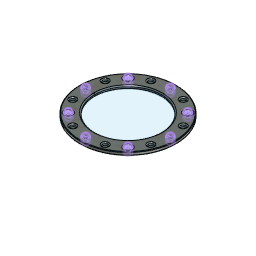
80mm-Gasket (Autodesk Fusion 360 design; units mm, degrees)
Autodesk Fusion 360 part; units mm, degrees
note: some values were not read from the file. Set by a fixed rule: which sketch regions a step uses.
sketch "Sketch1" plane through (0, 0, -3) normal (0, 0, -1) x (1, 0, 0)
  circle A0 centre (0, 0) radius 57.9733
  arc A1 (-37.591, -37.591) -> (-34.409, -34.409) centre (-36, -36) ccw
  arc A2 (-37.591, 37.591) -> (-34.409, 34.409) centre (-36, 36) ccw
  arc A3 (37.591, 37.591) -> (34.409, 34.409) centre (36, 36) ccw
  arc A4 (37.591, -37.591) -> (34.409, -34.409) centre (36, -36) ccw
  spline S0 degree 3 poles (-40, 0) (-40, -6.463) (-38.4036, -12.9202) (-32.3924, -24.3347) (-27.9941, -29.2878) (-18.5638, -35.7844) (-13.8953, -37.8426) (-2.3688, -40.5075) (4.666, -40.3075) (14.8449, -37.3359) (18.3282, -35.755) (26.9944, -30.2237) (31.596, -25.3745) (37.2725, -15.3601) (38.9152, -10.5255) (40.5307, 0.9912) (39.7923, 7.7648) (35.8254, 18.4158) (33.3642, 22.5705) (26.205, 30.8483) (21.0525, 34.5704) (10.4898, 38.9549) (5.2459, 40) (-6.442, 40) (-12.8781, 38.4142) (-23.2056, 32.9962) (-27.346, 29.6555) (-34.0803, 21.597) (-36.6527, 16.8665) (-39.3955, 7.9995) (-40, 4) (-40, 0) knots -1 -1 -1 -1 -0.922853 -0.922853 -0.84601 -0.84601 -0.786161 -0.786161 -0.704794 -0.704794 -0.659587 -0.659587 -0.582074 -0.582074 -0.522181 -0.522181 -0.443257 -0.443257 -0.386513 -0.386513 -0.312619 -0.312619 -0.25 -0.25 -0.173105 -0.173105 -0.11079 -0.11079 -0.047746 -0.047746 0 0 0 0
  circle A5 centre (0, 0) radius 57.9733
  spline S1 degree 3 poles (-40, 0) (-40, -6.463) (-38.4036, -12.9202) (-32.3924, -24.3347) (-27.9941, -29.2878) (-18.5638, -35.7844) (-13.8953, -37.8426) (-2.3688, -40.5075) (4.666, -40.3075) (14.8449, -37.3359) (18.3282, -35.755) (26.9944, -30.2237) (31.596, -25.3745) (37.2725, -15.3601) (38.9152, -10.5255) (40.5307, 0.9912) (39.7923, 7.7648) (35.8254, 18.4158) (33.3642, 22.5705) (26.205, 30.8483) (21.0525, 34.5704) (10.4898, 38.9549) (5.2459, 40) (-6.442, 40) (-12.8781, 38.4142) (-23.2056, 32.9962) (-27.346, 29.6555) (-34.0803, 21.597) (-36.6527, 16.8665) (-39.3955, 7.9995) (-40, 4) (-40, 0) knots -1 -1 -1 -1 -0.922853 -0.922853 -0.84601 -0.84601 -0.786161 -0.786161 -0.704794 -0.704794 -0.659587 -0.659587 -0.582074 -0.582074 -0.522181 -0.522181 -0.443257 -0.443257 -0.386513 -0.386513 -0.312619 -0.312619 -0.25 -0.25 -0.173105 -0.173105 -0.11079 -0.11079 -0.047746 -0.047746 0 0 0 0
  arc A6 (-37.591, 37.591) -> (-34.409, 34.409) centre (-36, 36) ccw construction
  arc A7 (37.591, 37.591) -> (34.409, 34.409) centre (36, 36) ccw construction
  circle A8 centre (36, -36) radius 2.1 construction
  arc A9 (-37.591, -37.591) -> (-34.409, -34.409) centre (-36, -36) ccw construction
  circle A10 centre (-36, 36) radius 2.25
  circle A11 centre (36, 36) radius 2.25
  circle A12 centre (36, -36) radius 2.25
  circle A13 centre (-36, -36) radius 2.25
  circle A14 centre (-51, 0) radius 2.25
  circle A15 centre (0, -51) radius 2.25
  circle A16 centre (51, 0) radius 2.25
  circle A17 centre (0, 51) radius 2.25
  dimension "d74" = 4.5
  dimension "d75" = 4.5
  dimension "d76" = 4.5
  dimension "d77" = 4.5
  dimension "d84" = 4.5
  dimension "d85" = 4.5
  dimension "d86" = 4.5
  dimension "d87" = 4.5
  constraint concentric A6 A10
  constraint concentric A7 A11
  constraint concentric A8 A12
  constraint concentric A9 A13
  measures "d74" diameter of A10
  measures "d75" diameter of A11
  measures "d76" diameter of A12
  measures "d77" diameter of A13
  measures "d84" diameter of A14
  measures "d85" diameter of A15
  measures "d86" diameter of A16
  measures "d87" diameter of A17
extrude "Extrude1" add sketch "Sketch1" along normal blind 4
sketch "Sketch2" plane through (0, 0, -3) normal (0, 0, 1) x (-1, 0, 0)
  spline S0 degree 3 poles (40, 0) (40, 4) (39.3955, 7.9995) (36.6527, 16.8665) (34.0803, 21.597) (27.346, 29.6555) (23.2056, 32.9962) (12.8781, 38.4142) (6.442, 40) (-5.2459, 40) (-10.4898, 38.9549) (-21.0525, 34.5704) (-26.205, 30.8483) (-33.3642, 22.5705) (-35.8254, 18.4158) (-39.7923, 7.7648) (-40.5307, 0.9912) (-38.9152, -10.5255) (-37.2725, -15.3601) (-31.596, -25.3745) (-26.9944, -30.2237) (-18.3282, -35.755) (-14.8449, -37.3359) (-4.666, -40.3075) (2.3688, -40.5075) (13.8953, -37.8426) (18.5638, -35.7844) (27.9941, -29.2878) (32.3924, -24.3347) (38.4036, -12.9202) (40, -6.463) (40, 0) knots 0 0 0 0 0.047746 0.047746 0.11079 0.11079 0.173105 0.173105 0.25 0.25 0.312619 0.312619 0.386513 0.386513 0.443257 0.443257 0.522181 0.522181 0.582074 0.582074 0.659587 0.659587 0.704794 0.704794 0.786161 0.786161 0.84601 0.84601 0.922853 0.922853 1 1 1 1
  circle A0 centre (0, 0) radius 57.9733
  circle A1 centre (0, -51) radius 2.25
  circle A2 centre (51, 0) radius 2.25
  circle A3 centre (0, 51) radius 2.25
  circle A4 centre (-51, 0) radius 2.25
  circle A5 centre (-36, -36) radius 2.25
  circle A6 centre (36, -36) radius 2.25
  circle A7 centre (36, 36) radius 2.25
  circle A8 centre (-36, 36) radius 2.25
sketch "Sketch3" plane through (0, 0, -7) normal (0, 0, -1) x (1, 0, 0)
  spline S0 degree 3 poles (-40, 0) (-40, 4) (-39.3955, 7.9995) (-36.6527, 16.8665) (-34.0803, 21.597) (-27.346, 29.6555) (-23.2056, 32.9962) (-12.8781, 38.4142) (-6.442, 40) (5.2459, 40) (10.4898, 38.9549) (21.0525, 34.5704) (26.205, 30.8483) (33.3642, 22.5705) (35.8254, 18.4158) (39.7923, 7.7648) (40.5307, 0.9912) (38.9152, -10.5255) (37.2725, -15.3601) (31.596, -25.3745) (26.9944, -30.2237) (18.3282, -35.755) (14.8449, -37.3359) (4.666, -40.3075) (-2.3688, -40.5075) (-13.8953, -37.8426) (-18.5638, -35.7844) (-27.9941, -29.2878) (-32.3924, -24.3347) (-38.4036, -12.9202) (-40, -6.463) (-40, 0) knots 0 0 0 0 0.047746 0.047746 0.11079 0.11079 0.173105 0.173105 0.25 0.25 0.312619 0.312619 0.386513 0.386513 0.443257 0.443257 0.522181 0.522181 0.582074 0.582074 0.659587 0.659587 0.704794 0.704794 0.786161 0.786161 0.84601 0.84601 0.922853 0.922853 1 1 1 1
  circle A0 centre (0, 0) radius 57.9733
  circle A1 centre (0, -51) radius 2.25
  circle A2 centre (-51, 0) radius 2.25
  circle A3 centre (0, 51) radius 2.25
  circle A4 centre (51, 0) radius 2.25
  circle A5 centre (36, -36) radius 2.25
  circle A6 centre (-36, -36) radius 2.25
  circle A7 centre (-36, 36) radius 2.25
  circle A8 centre (36, 36) radius 2.25
sketch "Sketch4" plane through (0, 0, -3) normal (0, 0, 1) x (-1, 0, 0)
  circle A0 centre (-36, -36) radius 3.75
  circle A1 centre (36, -36) radius 3.75
  circle A2 centre (36, 36) radius 3.75
  circle A3 centre (-36, 36) radius 3.75
  dimension "d78" = 7.5
  dimension "d79" = 7.5
  dimension "d80" = 7.5
  dimension "d81" = 7.5
  measures "d78" diameter of A0
  measures "d79" diameter of A1
  measures "d80" diameter of A2
  measures "d81" diameter of A3
chamfer "Chamfer2" distance 3 angle 45 4 edges at (33.9023, -36.8136, -3) (-38.0977, -36.8136, -3) (33.9023, 35.1864, -3) (-38.0977, 35.1864, -3)
chamfer "Chamfer3" distance 3 angle 45 4 edges at (48.9023, -0.8136, -7) (-2.0977, -51.8136, -7) (-53.0977, -0.8136, -7) (-2.0977, 50.1864, -7)
chamfer "Chamfer4" distance 1.2 angle 45 2 edges at (39.9959, 0.0004, -3) (39.9959, 0.0004, -7)
chamfer "Chamfer5" distance 0.6 angle 45 2 edges at (-54.0501, 20.964, -7) (-54.0501, 20.964, -3)
sketch "Sketch5" plane through (0, 0, -3) normal (0, 0, 1) x (1, 0, 0)
  line L0 (0, 0) -> (84.9266, 35.1777) construction
  line L1 (0, 0) -> (91.9239, 0) construction
  circle A0 centre (0, 0) radius 50.9117 construction
  line L2 (0, 0) -> (100, 0) construction
  line L3 (0, 0) -> (-91.4454, -37.8779) construction
  line L4 (0, 0) -> (98.9798, 0) construction
  line L5 (0, 0) -> (-3, 3) construction
  line L6 (0, 0) -> (29.4964, -71.2107) construction
  line L7 (0, 0) -> (77.0779, 0) construction
  line L8 (0, 0) -> (29.6754, 71.6428) construction
  line L9 (0, 0) -> (-77.5456, 0) construction
  line L10 (0, 0) -> (68.8989, -28.5389) construction
  line L11 (0, 0) -> (-74.5757, 0) construction
  line L12 (67.0262, -27.7632) -> (-71.3068, 29.5363) construction
  line L13 (13.5342, -32.6745) -> (-28.434, 68.6458) construction
  circle A1 centre (47.0363, -19.4831) radius 3.1
  circle A2 centre (47.0363, 19.4831) radius 3.1
  line L14 (0, -67) -> (0, 85) construction
  circle A3 centre (-47.0363, -19.4831) radius 3.1
  circle A4 centre (-47.0363, 19.4831) radius 3.1
  circle A5 centre (-19.4831, 47.0363) radius 3.1
  circle A6 centre (-19.4831, -47.0363) radius 3.1
  circle A7 centre (-47.0363, -19.4831) radius 3.1
  circle A8 centre (19.4831, 47.0363) radius 3.1
  circle A9 centre (19.4831, -47.0363) radius 3.1
  dimension "d4" = 22.5
  dimension "d5" = 91.9239
  dimension "d8" = 157.5
  dimension "d9" = 67.5
  dimension "d10" = 112.5
  dimension "d11" = 157.5
  dimension "d12" = 6.2
  dimension "d17" = 6.2
  constraint horizontal L1
  constraint coincident L0.start L1.start
  constraint horizontal L2
  constraint horizontal L4
  constraint horizontal L7
  constraint horizontal L9
  constraint horizontal L11
  constraint coincident L10 L12.start
  constraint parallel L10 L12
  constraint coincident L6 L13.start
  constraint perpendicular L0 L13
  constraint coincident A0 A1.centre
  constraint coincident L12 A1.centre
  constraint symmetric L1 A1 A2
  constraint vertical L14
  constraint symmetric A1 L14 A3
  constraint symmetric A2 L14 A4
  constraint coincident A0 A5.centre
  constraint coincident L13 A5.centre
  constraint symmetric L9 A5 A6
  constraint symmetric A1 L14 A7
  constraint symmetric L14 A5 A8
  constraint symmetric L14 A6 A9
  measures "d4" angle of L0 L1
  measures "d5" distance of L0.start L0.end
  measures "d8" angle of L3 L4
  measures "d9" angle of L6 L7
  measures "d10" angle of L8 L9
  measures "d11" angle of L10 L11
  measures "d12" diameter of A1
  measures "d17" diameter of A5
extrude "Extrude3" cut sketch "Sketch5" against normal up to surface (3 mm away)
chamfer "Chamfer6" distance 1.2 angle 45 8 edges at (44.1461, -18.3621, -3) (44.1461, 20.6041, -3) (-49.9265, -18.3621, -3) (-49.9265, 20.6041, -3) (16.5928, -45.9153, -3) (-22.3733, -45.9153, -3) (-22.3733, 48.1573, -3) (16.5928, 48.1573, -3)
equation "d74 = baseScrewHoleDiameter"
equation "d75 = baseScrewHoleDiameter"
equation "d76 = baseScrewHoleDiameter"
equation "d77 = baseScrewHoleDiameter"
equation "d84 = baseScrewHoleDiameter"
equation "d85 = baseScrewHoleDiameter"
equation "d86 = baseScrewHoleDiameter"
equation "d87 = baseScrewHoleDiameter"
equation "baseScrewHoleDiameter = 4.5 mm" comment "Holes / slot spacing for base ring holes"
equation "d12 = magnetHoleSize"
equation "magnetHoleSize = 6.2 mm"
equation "d17 = magnetHoleSize"
